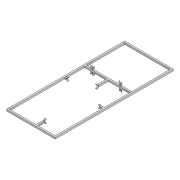
# Autodesk Inventor part: Pieza2
Saved by Autodesk Inventor 2021 (Build 250183000, 183)
## iProperties
Created: 2021-07-10
Part Number: Pieza2
Material: Genérico
Document SubType Name: Modeling
Designer: Admin
Density: 1 g/cm^3
Appearance: Valor por defecto
Author: Admin
Autodesk Inventor part; units mm, degrees
ref_plane "YZ Plane" through (0, 0, 0) normal (1, 0, 0) x (0, 1, 0)
ref_plane "XZ Plane" through (0, 0, 0) normal (0, 1, 0) x (-1, 0, 0)
ref_plane "XY Plane" through (0, 0, 0) normal (0, 0, 1) x (1, 0, 0)
sketch "Boceto1" plane through (0, 0, 0) normal (1, 0, 0) x (0, 1, 0)
  line L0 (0, 0) -> (20, 0)
  line L1 (20, 0) -> (20, -20)
  line L2 (20, -20) -> (0, -20)
  line L3 (0, -20) -> (0, 0)
  dimension "d0" = 20
  dimension "d1" = 20
  constraints: 8 end point, 2 parallel, 1 horizontal, 1 perpendicular
  measures "d0" distance of L1.end L2.end
  measures "d1" distance of L0.end L1.end
extrude "Extrusión1" add sketch "Boceto1" along normal blind 624
sketch "Boceto2" plane through (0, 0, 0) normal (0, 0, 1) x (1, 0, 0)
  point P0 (0, 0)
sketch "Boceto3" plane through (0, 0, 0) normal (0, 0, 1) x (1, 0, 0)
  line L0 (0, 20.2367) -> (20, 20.2367)
  line L1 (20, 20.2367) -> (20, 0.2367)
  line L2 (20, 0.2367) -> (0, 0.2367)
  line L3 (0, 0.2367) -> (0, 20.2367)
  line L4 (0, 0) -> (624, 0) projected
  line L5 (624, 0) -> (604, 0)
  line L6 (604, 0) -> (604, 20)
  line L7 (604, 20) -> (624, 20)
  line L8 (624, 20) -> (624, 0)
  dimension "d4" = 20
  dimension "d5" = 20
  dimension "d6" = 20
  dimension "d7" = 20
  constraints: 16 end point, 4 parallel, 2 horizontal, 2 perpendicular
  measures "d4" distance of L1.end L2.end
  measures "d5" distance of L0.end L1.end
  measures "d6" distance of L6.end L7.end
  measures "d7" distance of L5.end L6.end
extrude "Extrusión2" add sketch "Boceto3" along normal blind 1470
sketch "Boceto4" plane through (0, 0, 1470) normal (0, 0, 1) x (1, 0, 0)
  line L0 (624, 0) -> (624, 20) projected
  line L1 (0, 0) -> (604, 0) projected
  line L2 (624, 20) -> (0, 20)
  line L3 (0, 20) -> (0, 0)
  line L4 (0, 0) -> (624, 0)
  line L5 (624, 0) -> (624, 20)
  constraints: 8 end point, 2 parallel, 1 horizontal, 1 perpendicular
extrude "Extrusión3" add sketch "Boceto4" along normal blind 20
sketch "Boceto5" plane through (20, 20.2367, 1470) normal (1, 0, 0) x (0, 0, -1)
  line L0 (1470, 0) -> (0, 0) projected
  line L1 (956.7483, 0) -> (976.7483, 0)
  line L2 (976.7483, 0) -> (976.7483, -20)
  line L3 (976.7483, -20) -> (956.7483, -20)
  line L4 (956.7483, -20) -> (956.7483, 0)
  point P0 (1470, -20.2367)
  dimension "d12" = 20
  dimension "d13" = 20
  constraints: 8 end point, 2 parallel, 1 horizontal, 1 perpendicular, 1 point on line
  measures "d12" distance of L2.end L3.end
  measures "d13" distance of L1.end L2.end
extrude "Extrusión4" add sketch "Boceto5" along normal blind 584
sketch "Boceto6" plane through (0, 0, 1470) normal (0, 0, -1) x (-1, 0, 0)
  line L0 (-604, 20) -> (-20, 20) projected
  line L1 (-604, 20) -> (-377, 20)
  line L2 (-377, 20) -> (-357, 20)
  line L3 (-357, 20) -> (-357, 0)
  line L4 (-357, 0) -> (-377, 0)
  line L5 (-377, 0) -> (-377, 20)
  point P0 (0, 0)
  dimension "d16" = 227
  dimension "d17" = 20
  dimension "d18" = 20
  constraints: 10 end point, 2 parallel, 1 horizontal, 1 perpendicular, 1 point on line
  measures "d16" distance of L0.start L1.end
  measures "d17" distance of L3.end L4.end
  measures "d18" distance of L2.end L3.end
extrude "Extrusión5" add sketch "Boceto6" along normal blind 90.6
sketch "Boceto7" plane through (377, 0, 1470) normal (1, 0, 0) x (0, 0, -1)
  arc A0 (114.9903, 31.082) -> (114.9903, -11.082) centre (114.9903, 10) ccw
  arc A1 (114.9903, 34.3903) -> (114.9903, -14.3903) centre (114.9903, 10) ccw
  line L0 (114.9903, 34.3903) -> (114.9903, 31.082)
  line L1 (114.9903, -11.082) -> (114.9903, -14.3903)
  point P0 (1470, 0)
  dimension "d21" = 42.164
  constraints: 4 end point, 4 point on circle, 2 centre point, 2 vertical, 1 coincident
  measures "d21" diameter of A0
extrude "Extrusión6" add sketch "Boceto7" against normal blind 20
sketch "Boceto8" plane through (0, 20.2367, 1470) normal (0, 1, 0) x (1, 0, 0)
  line L0 (20, 956.7483) -> (604, 956.7483) projected
  line L1 (20, 956.7483) -> (97.615, 956.7483)
  line L2 (20, 976.7483) -> (604, 976.7483) projected
  line L3 (20, 976.7483) -> (104.527, 976.7483)
  line L4 (104.527, 976.7483) -> (97.615, 956.7483)
  line L5 (97.615, 956.7483) -> (117.615, 956.7483)
  line L6 (117.615, 956.7483) -> (124.527, 976.7483)
  line L7 (104.527, 976.7483) -> (124.527, 976.7483)
  line L8 (604, 956.7483) -> (484.073, 956.7483)
  line L9 (604, 976.7483) -> (604, 956.7483) projected
  line L10 (604, 976.7483) -> (474.073, 976.7483)
  line L11 (20, 976.7483) -> (604, 976.7483) projected
  line L12 (484.073, 956.7483) -> (474.073, 976.7483)
  line L13 (474.073, 976.7483) -> (454.073, 976.7483)
  line L14 (484.073, 956.7483) -> (464.073, 956.7483)
  line L15 (464.073, 956.7483) -> (454.073, 976.7483)
  point P0 (0, 1470)
  dimension "d24" = 77.615
  dimension "d25" = 84.527
  dimension "d26" = 20
  dimension "d27" = 119.927
  dimension "d28" = 129.927
  dimension "d29" = 20
  dimension "d30" = 20
  constraints: 24 end point, 8 point on line, 1 collinear, 1 parallel
  measures "d24" distance of L0.start L1.end
  measures "d25" distance of L2.start L3.end
  measures "d26" distance of L1.end L5.end
  measures "d27" distance of L0.end L8.end
  measures "d28" distance of L2.end L10.end
  measures "d29" distance of L10.end L13.end
  measures "d30" distance of L8.end L14.end
extrude "Extrusión7" add sketch "Boceto8" along normal blind 20 contours L4 L2 L6 L0
sketch "Boceto10" plane through (20, 0.2367, 493.2517) normal (0, 0, -1) x (-1, 0, 0)
  arc A0 (-109.3817, 55.7334) -> (-79.3817, 55.7334) centre (-94.3817, 55.7334) ccw
  arc A1 (-110.8817, 55.7334) -> (-77.8817, 55.7334) centre (-94.3817, 55.7334) ccw
  line L0 (-110.8817, 55.7334) -> (-109.3817, 55.7334)
  line L1 (-79.3817, 55.7334) -> (-77.8817, 55.7334)
  point P0 (20, -0.2367)
  dimension "d33" = 30
  dimension "d36" = 33
  constraints: 4 end point, 4 point on circle, 2 centre point, 2 point on line, 1 coincident, 1 horizontal
  measures "d33" diameter of A0
  measures "d36" diameter of A1
sketch "Boceto11" plane through (20, 0.2367, 513.2517) normal (0, 0, 1) x (1, 0, 0)
  arc A0 (73.8257, 55.7334) -> (103.8257, 55.7334) centre (88.8257, 55.7334) ccw
  arc A1 (72.3257, 55.7334) -> (105.3257, 55.7334) centre (88.8257, 55.7334) ccw
  line L0 (73.8257, 55.7334) -> (72.3257, 55.7334)
  line L1 (103.8257, 55.7334) -> (105.3257, 55.7334)
  point P0 (-20, -0.2367)
  dimension "d34" = 30
  dimension "d35" = 33
  constraints: 4 end point, 4 point on circle, 2 centre point, 2 point on line, 1 coincident, 1 horizontal
  measures "d34" diameter of A0
  measures "d35" diameter of A1
loft "Solevación1" add profiles "Boceto10", "Boceto11"
sketch "Boceto12" plane through (0, 0.2367, 0) normal (0, -1, 0) x (1, 0, 0)
  line L0 (20, 513.2517) -> (604, 513.2517) projected
  line L1 (20, 513.2517) -> (97.615, 513.2517)
  line L2 (19.9998, 493.2517) -> (104.527, 493.2517)
  line L3 (20, 493.2517) -> (104.527, 493.2517) projected
  line L4 (104.527, 493.2517) -> (97.615, 513.2517)
  line L5 (113.7965, 513.2517) -> (117.615, 513.2517) projected
  line L6 (97.615, 513.2517) -> (117.615, 513.2517)
  line L7 (117.615, 513.2517) -> (124.527, 493.2517) projected
  line L8 (117.615, 513.2517) -> (124.527, 493.2517)
  line L9 (124.527, 493.2517) -> (104.527, 493.2517)
  point P0 (0, 0)
  dimension "d41" = 77.615
  constraints: 12 end point, 2 collinear, 2 horizontal, 1 point on line
  measures "d41" distance of L0.start L1.end
extrude "Extrusión8" add sketch "Boceto12" along normal blind 20
sketch "Boceto13" plane through (20, 0.2367, 513.2517) normal (0, 0, 1) x (1, 0, 0)
  arc A0 (102.615, -36.243) -> (72.615, -36.243) centre (87.615, -36.243) ccw
  arc A1 (104.115, -36.243) -> (71.115, -36.243) centre (87.615, -36.243) ccw
  line L0 (104.115, -36.243) -> (102.615, -36.243)
  line L1 (72.615, -36.243) -> (71.115, -36.243)
  point P0 (-20, -0.2367)
  dimension "d44" = 30
  dimension "d45" = 33
  constraints: 4 end point, 4 point on circle, 2 centre point, 2 point on line, 1 coincident, 1 horizontal
  measures "d44" diameter of A0
  measures "d45" diameter of A1
sketch "Boceto14" plane through (20, 0.2367, 493.2517) normal (0, 0, -1) x (-1, 0, 0)
  arc A0 (-79.527, -36.243) -> (-109.527, -36.243) centre (-94.527, -36.243) ccw
  arc A1 (-78.027, -36.243) -> (-111.027, -36.243) centre (-94.527, -36.243) ccw
  line L0 (-78.027, -36.243) -> (-79.527, -36.243)
  line L1 (-109.527, -36.243) -> (-111.027, -36.243)
  point P0 (20, -0.2367)
  point P1 (-87.615, -36.243)
  dimension "d46" = 30
  dimension "d47" = 33
  constraints: 4 end point, 4 point on circle, 2 centre point, 2 point on line, 1 coincident, 1 horizontal
  measures "d46" diameter of A0
  measures "d47" diameter of A1
loft "Solevación2" add profiles "Boceto14", "Boceto13"
sketch "Boceto15" plane through (604, 20.2367, 513.2517) normal (0, 1, 0) x (1, 0, 0)
  line L0 (-479.473, 20) -> (0, 20) projected
  line L1 (0, 20) -> (-129.927, 20)
  line L2 (0, 513.2517) -> (0, -956.7483) projected
  line L3 (0, -0.5168) -> (-119.927, -0.5168)
  line L4 (0, -0.5168) -> (119.927, -0.5168) construction
  line L5 (-119.927, -0.5168) -> (-129.927, 20)
  line L6 (-129.927, 20) -> (-149.927, 20)
  line L7 (-149.927, 20) -> (-140.1789, 0)
  line L8 (-486.385, 0) -> (0, 0) projected
  line L9 (-140.1789, 0) -> (-119.927, -0.5168)
  point P0 (-604, 513.2517)
  point P1 (-120.1789, 0)
  dimension "d52" = 129.927
  dimension "d53" = 119.927
  dimension "d54" = 180
  dimension "d55" = 20
  constraints: 14 end point, 4 point on line, 1 collinear, 1 horizontal, 1 parallel, 1 perpendicular
  measures "d52" distance of L0.end L1.end
  measures "d53" distance of L3.start L3.end
  measures "d54" angle of L3 L4
  measures "d55" distance of L1.end L6.end
extrude "Extrusión9" add sketch "Boceto15" along normal blind 25 contours L0 L5 L8 L7
sketch "Boceto16" plane through (20, 0.2367, 513.2517) normal (0, 0, 1) x (1, 0, 0)
  arc A0 (438.8211, 61.1945) -> (468.8211, 61.1945) centre (453.8211, 61.1945) ccw
  arc A1 (437.3211, 61.1945) -> (470.3211, 61.1945) centre (453.8211, 61.1945) ccw
  line L0 (437.3211, 61.1945) -> (438.8211, 61.1945)
  line L1 (-20, 19.7633) -> (604, 19.7633) projected
  line L2 (468.8211, 61.1945) -> (470.3211, 61.1945)
  point P0 (-20, -0.2367)
  dimension "d58" = 30
  dimension "d59" = 33
  constraints: 4 end point, 4 point on circle, 2 centre point, 1 coincident, 1 parallel, 1 point on line
  measures "d58" diameter of A0
  measures "d59" diameter of A1
sketch "Boceto17" plane through (20, 0.2367, 493.2517) normal (0, 0, -1) x (-1, 0, 0)
  arc A0 (-458.8211, 61.1945) -> (-428.8211, 61.1945) centre (-443.8211, 61.1945) ccw
  arc A1 (-460.3211, 61.1945) -> (-427.3211, 61.1945) centre (-443.8211, 61.1945) ccw
  line L0 (-460.3211, 61.1945) -> (-458.8211, 61.1945)
  line L1 (-428.8211, 61.1945) -> (-427.3211, 61.1945)
  point P0 (20, -0.2367)
  point P1 (-453.8211, 61.1945)
  dimension "d60" = 30
  dimension "d61" = 33
  constraints: 4 end point, 4 point on circle, 2 centre point, 2 point on line, 1 coincident, 1 horizontal
  measures "d60" diameter of A0
  measures "d61" diameter of A1
loft "Solevación3" add profiles "Boceto17", "Boceto16"
sketch "Boceto18" plane through (604, 0.2367, 493.2517) normal (0, -1, 0) x (1, 0, 0)
  line L0 (-479.473, 0) -> (0, 0) projected
  line L1 (0, 0) -> (-129.927, 0)
  line L2 (-486.385, 20) -> (0, 20) projected
  line L3 (0, 20) -> (-119.927, 20)
  line L4 (-119.927, 20) -> (-129.927, 0)
  line L5 (-129.927, 0) -> (-149.927, 0)
  line L6 (-486.385, 20) -> (-140.1789, 20) projected
  line L7 (-149.927, 0) -> (-140.1789, 20)
  line L8 (-140.1789, 20) -> (-119.927, 20)
  point P0 (-604, -493.2517)
  dimension "d66" = 129.927
  dimension "d67" = 119.927
  dimension "d68" = 20
  constraints: 12 end point, 3 point on line, 1 collinear
  measures "d66" distance of L0.end L1.end
  measures "d67" distance of L2.end L3.end
  measures "d68" distance of L1.end L5.end
extrude "Extrusión10" add sketch "Boceto18" along normal blind 25
sketch "Boceto19" plane through (20, 0.2367, 493.2517) normal (0, 0, -1) x (-1, 0, 0)
  arc A0 (-429.073, -41.0242) -> (-459.073, -41.0242) centre (-444.073, -41.0242) ccw
  arc A1 (-427.573, -41.0242) -> (-460.573, -41.0242) centre (-444.073, -41.0242) ccw
  line L0 (-427.573, -41.0242) -> (-429.073, -41.0242)
  line L1 (-459.073, -41.0242) -> (-460.573, -41.0242)
  point P0 (20, -0.2367)
  dimension "d71" = 30
  dimension "d72" = 33
  constraints: 4 end point, 4 point on circle, 2 centre point, 2 point on line, 1 coincident, 1 horizontal
  measures "d71" diameter of A0
  measures "d72" diameter of A1
sketch "Boceto20" plane through (20, 0.2367, 513.2517) normal (0, 0, 1) x (1, 0, 0)
  arc A0 (469.073, -41.0242) -> (439.073, -41.0242) centre (454.073, -41.0242) ccw
  arc A1 (470.573, -41.0242) -> (437.573, -41.0242) centre (454.073, -41.0242) ccw
  line L0 (470.573, -41.0242) -> (469.073, -41.0242)
  line L1 (439.073, -41.0242) -> (437.573, -41.0242)
  point P0 (-20, -0.2367)
  point P1 (444.073, -41.0242)
  dimension "d73" = 30
  dimension "d74" = 33
  constraints: 4 end point, 4 point on circle, 2 centre point, 2 point on line, 1 coincident, 1 horizontal
  measures "d73" diameter of A0
  measures "d74" diameter of A1
loft "Solevación4" add profiles "Boceto20", "Boceto19"
sketch "Boceto21" plane through (20, 0.2367, 513.2517) normal (0, 0, 1) x (1, 0, 0)
  line L0 (97.615, 0) -> (443.8211, 0) projected
  line L1 (97.615, 20) -> (443.8211, 20) projected
  line L2 (305.0225, 0) -> (285.0225, 0)
  line L3 (285.0225, 0) -> (285.0225, 20)
  line L4 (285.0225, 20) -> (305.0225, 20)
  line L5 (305.0225, 20) -> (305.0225, 0)
  point P0 (-20, -0.2367)
  dimension "d79" = 20
  dimension "d80" = 20
  constraints: 8 end point, 2 parallel, 1 horizontal, 1 perpendicular, 1 point on line
  measures "d79" distance of L3.end L4.end
  measures "d80" distance of L2.end L3.end
extrude "Extrusión11" add sketch "Boceto21" along normal blind 124
sketch "Boceto22" plane through (325.0225, 0.2367, 513.2517) normal (1, 0, 0) x (0, 0, -1)
  arc A0 (-147.0775, -10.3944) -> (-147.0775, 32.6056) centre (-147.0775, 11.1056) ccw
  arc A1 (-147.0775, -12.3944) -> (-147.0775, 34.6056) centre (-147.0775, 11.1056) ccw
  line L0 (-147.0775, -12.3944) -> (-147.0775, -10.3944)
  line L1 (-147.0775, 32.6056) -> (-147.0775, 34.6056)
  point P0 (513.2517, -0.2367)
  dimension "d83" = 43
  dimension "d84" = 47
  constraints: 4 end point, 4 point on circle, 2 centre point, 2 point on line, 1 coincident, 1 vertical
  measures "d83" diameter of A0
  measures "d84" diameter of A1
extrude "Extrusión12" add sketch "Boceto22" against normal blind 20
sketch "Boceto23" plane through (604, 0, 0) normal (-1, 0, 0) x (0, 0, 1)
  line L0 (513.2517, 20) -> (1470, 20) projected
  line L1 (0, 0) -> (1470, 0) projected
  line L2 (845.6815, 20) -> (865.6815, 20)
  line L3 (865.6815, 20) -> (865.6815, 0)
  line L4 (865.6815, 0) -> (845.6815, 0)
  line L5 (845.6815, 0) -> (845.6815, 20)
  dimension "d87" = 20
  dimension "d88" = 20
  constraints: 8 end point, 2 parallel, 1 horizontal, 1 perpendicular, 1 point on line
  measures "d87" distance of L3.end L4.end
  measures "d88" distance of L2.end L3.end
extrude "Extrusión13" add sketch "Boceto23" along normal blind 39
sketch "Boceto24" plane through (604, 0, 845.6815) normal (0, 0, -1) x (-1, 0, 0)
  arc A0 (57.4695, 27.5) -> (57.4695, -7.5) centre (57.4695, 10) ccw
  arc A1 (57.4695, 29) -> (57.4695, -9) centre (57.4695, 10) ccw
  line L0 (57.4695, 29) -> (57.4695, 27.5)
  line L1 (57.4695, -7.5) -> (57.4695, -9)
  point P0 (604, 0)
  dimension "d91" = 35
  dimension "d92" = 38
  constraints: 4 end point, 4 point on circle, 2 centre point, 2 point on line, 1 coincident, 1 vertical
  measures "d91" diameter of A0
  measures "d92" diameter of A1
extrude "Extrusión14" add sketch "Boceto24" against normal blind 20
sketch "Boceto25" plane through (20, 0.2367, 1470) normal (1, 0, 0) x (0, 0, -1)
  line L0 (704.3678, 19.8141) -> (724.3678, 19.8141)
  line L1 (724.3678, 19.8141) -> (724.3678, -0.1859)
  line L2 (724.3678, -0.1859) -> (704.3678, -0.1859)
  line L3 (704.3678, -0.1859) -> (704.3678, 19.8141)
  point P0 (1470, -0.2367)
  dimension "d95" = 20
  dimension "d96" = 20
  constraints: 8 end point, 2 parallel, 1 horizontal, 1 perpendicular
  measures "d95" distance of L1.end L2.end
  measures "d96" distance of L0.end L1.end
extrude "Extrusión15" add sketch "Boceto25" along normal blind 18
sketch "Boceto26" plane through (20, 0.2367, 765.6322) normal (0, 0, 1) x (1, 0, 0)
  arc A0 (36.5801, 27.3141) -> (36.5801, -7.6859) centre (36.5801, 9.8141) ccw
  arc A1 (36.5801, 28.8141) -> (36.5801, -9.1859) centre (36.5801, 9.8141) ccw
  line L0 (36.5801, 28.8141) -> (36.5801, 27.3141)
  line L1 (36.5801, -7.6859) -> (36.5801, -9.1859)
  point P0 (-20, -0.2367)
  dimension "d99" = 35
  dimension "d100" = 38
  constraints: 4 end point, 4 point on circle, 2 centre point, 2 point on line, 1 coincident
  measures "d99" diameter of A0
  measures "d100" diameter of A1
extrude "Extrusión16" add sketch "Boceto26" against normal blind 20
